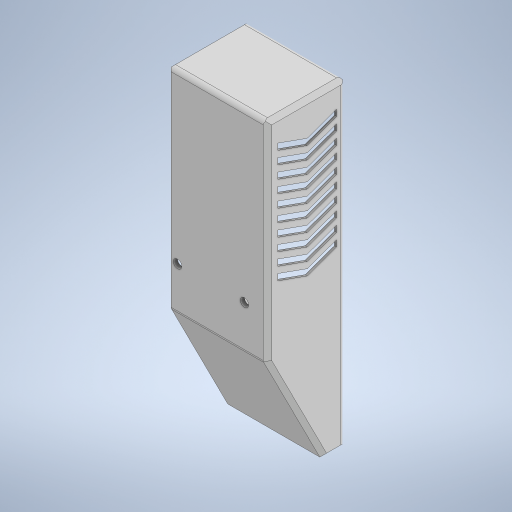
# Autodesk Inventor part: LewyBłotnik
Saved by Autodesk Inventor 2024 (Build 280153000, 153)
## iProperties
Created: 2025-05-22
Part Number: LewyBłotnik
Material: Ogólny
Document SubType Name: Modeling
Designer: Victoria
Density: 1 g/cm^3
Appearance: Domyślna
Author: Victoria
Autodesk Inventor part; units mm, degrees
ref_plane "YZ Plane" through (0, 0, 0) normal (1, 0, 0) x (0, 1, 0)
ref_plane "XZ Plane" through (0, 0, 0) normal (0, 1, 0) x (-1, 0, 0)
ref_plane "XY Plane" through (0, 0, 0) normal (0, 0, 1) x (1, 0, 0)
sketch "Szkic1" plane through (0, 0, 0) normal (0, 0, 1) x (1, 0, 0)
  circle A0 centre (16, 0) radius 2
  circle A1 centre (-16, 0) radius 2
  line L0 (28, -73) -> (-21, -73)
  line L1 (-21, -73) -> (-21, 0)
  line L2 (28, 80) -> (-21, 80)
  line L3 (-21, 80) -> (-21, 0)
  line L4 (28, -73) -> (27, -73)
  line L5 (27, -73) -> (27, 80)
  point P0 (0, 0)
  point P1 (-21, 83.4616)
  dimension "d0" = 4
  dimension "d48" = 1
  constraints: 12 end point, 3 perpendicular, 3 point on line, 2 centre point
  measures "d0" diameter of A0
  measures "d48" distance of L0.start L4.end
extrude "Wyciągnięcie proste1" add sketch "Szkic1" along normal blind 2
sketch "Szkic2" plane through (0, 0, 0) normal (0, 0, -1) x (-1, 0, 0)
  line L0 (21, -73) -> (-27, -73) projected
  line L1 (21, 80) -> (21, -73) projected
  circle A0 centre (16, 0) radius 2 projected
  circle A1 centre (-16, 0) radius 2 projected
  line L2 (19, -10) -> (21, -10)
  line L3 (-27, 80) -> (21, 80) projected
  line L4 (19, -71) -> (-26, -71)
  line L5 (-26, -71) -> (-26, 78)
  line L6 (-26, 78) -> (19, 78)
  line L7 (19, 78) -> (19, -71)
  line L8 (19, 68) -> (21, 68)
  line L9 (-27, -73) -> (-27, 80) projected
  point P0 (0, 0)
  dimension "d10" = 2
  constraints: 12 end point, 3 point on line, 2 perpendicular, 1 other
  measures "d10" distance between parallel lines of L1 L7
extrude "Wyciągnięcie proste2" add sketch "Szkic2" along normal blind 35 contours L0 L9 L3 L1 L8 L7 L6 L5 L4 L2 | L2 L7 L8 L1
sketch "Szkic7" plane through (27, -73, 2) normal (1, 0, 0) x (0, 0, -1)
  line L0 (0, 0) -> (0, 153) projected
  line L1 (37, 0) -> (0, 0) projected
  line L2 (0, 53) -> (27, 0) projected
  point P0 (2, 73)
extrude "Wyciągnięcie proste7" cut sketch "Szkic7" against normal up to surface (48 mm away)
sketch "Szkic9" plane through (27, -73, -35) normal (1, 0, 0) x (0, 0, -1)
  line L0 (-37, 53) -> (-10, 0) projected
  line L1 (0, 0) -> (-10, 0) projected
  line L2 (0, 153) -> (0, 0) projected
  line L3 (0, 153) -> (-37, 153) projected
  line L4 (-37, 53) -> (-37, 153) projected
  line L5 (-10, 0) -> (-8, 0)
  line L6 (0, 0) -> (-10, 0) projected
  line L7 (-37, 53) -> (-35, 53)
  line L8 (-35, 53) -> (-8, 0)
  point P0 (-35, 73)
  point P1 (-8, 0)
  dimension "d54" = 2
  dimension "d55" = 2
  constraints: 6 end point, 1 horizontal, 1 point on line
  measures "d54" distance of L0.end L5.end
  measures "d55" distance of L0.start L7.end
extrude "Wyciągnięcie proste9" add sketch "Szkic9" against normal up to surface (48 mm away) contours L7 L8 L1 L0
chamfer "Faza2" distance 2 angle 45 16 edges at (27, -46.5, -11.5) (27, -73, -30) (27, 30, 2) (27, 80, -16.5) (26, -45.5, -12.9906) (26, -71, -30.4906) (26, 29, 0) (26, 78, -17.5) (-21, -46.5, -11.5) (-21, -73, -30) (-21, 30, 2) (-21, 80, -16.5) (-19, 29, 0) (-19, -45.5, -12.9906) (-19, -71, -30.4906) (-19, 78, -17.5)
fillet "Zaokrąglenie2" radius 2 6 edges at (3, -73, -35) (3, 80, -35) (-21, 3.5, -35) (27, 3.5, -35) (3, -20, 2) (3, 80, 2)
sketch "Szkic13" plane through (27, -19.5199, 0) normal (1, 0, 0) x (0, 0, -1)
  line L0 (33, 97.5199) -> (33, 106.5199)
  line L1 (33, 106.5199) -> (17, 106.5199)
  line L2 (1, 106.5199) -> (33, 106.5199)
  line L3 (17, 106.5199) -> (17, 193.3833)
  line L4 (17, 106.5199) -> (17, 111.5199)
  line L5 (31, 106.5199) -> (17, 111.5199)
  line L6 (17, 111.5199) -> (3, 106.5199)
  line L7 (31, 106.5199) -> (31, 109.5199)
  line L8 (17, 111.5199) -> (17, 114.5199)
  line L9 (17, 114.5199) -> (31, 109.5199)
  line L10 (3, 106.5199) -> (3, 109.5199)
  line L11 (3, 193.7998) -> (3, 99.5199)
  line L12 (3, 109.5199) -> (17, 114.5199)
  line L13 (17, 117.5199) -> (3, 112.5199)
  line L14 (3, 115.5199) -> (17, 120.5199)
  line L15 (3, 112.5199) -> (3, 115.5199)
  line L16 (31, 112.5199) -> (17, 117.5199)
  line L17 (17, 120.5199) -> (31, 115.5199)
  line L18 (31, 112.5199) -> (31, 115.5199)
  line L19 (17, 123.5199) -> (3, 118.5199)
  line L20 (3, 121.5199) -> (17, 126.5199)
  line L21 (3, 118.5199) -> (3, 121.5199)
  line L22 (31, 118.5199) -> (17, 123.5199)
  line L23 (17, 126.5199) -> (31, 121.5199)
  line L24 (31, 118.5199) -> (31, 121.5199)
  line L25 (17, 129.5199) -> (3, 124.5199)
  line L26 (3, 127.5199) -> (17, 132.5199)
  line L27 (3, 124.5199) -> (3, 127.5199)
  line L28 (31, 124.5199) -> (17, 129.5199)
  line L29 (17, 132.5199) -> (31, 127.5199)
  line L30 (31, 124.5199) -> (31, 127.5199)
  line L31 (17, 135.5199) -> (3, 130.5199)
  line L32 (3, 133.5199) -> (17, 138.5199)
  line L33 (3, 130.5199) -> (3, 133.5199)
  line L34 (31, 130.5199) -> (17, 135.5199)
  line L35 (17, 138.5199) -> (31, 133.5199)
  line L36 (31, 130.5199) -> (31, 133.5199)
  line L37 (17, 141.5199) -> (3, 136.5199)
  line L38 (3, 139.5199) -> (17, 144.5199)
  line L39 (3, 136.5199) -> (3, 139.5199)
  line L40 (31, 136.5199) -> (17, 141.5199)
  line L41 (17, 144.5199) -> (31, 139.5199)
  line L42 (31, 136.5199) -> (31, 139.5199)
  line L43 (17, 147.5199) -> (3, 142.5199)
  line L44 (3, 145.5199) -> (17, 150.5199)
  line L45 (3, 142.5199) -> (3, 145.5199)
  line L46 (31, 142.5199) -> (17, 147.5199)
  line L47 (17, 150.5199) -> (31, 145.5199)
  line L48 (31, 142.5199) -> (31, 145.5199)
  line L49 (17, 153.5199) -> (3, 148.5199)
  line L50 (3, 151.5199) -> (17, 156.5199)
  line L51 (3, 148.5199) -> (3, 151.5199)
  line L52 (31, 148.5199) -> (17, 153.5199)
  line L53 (17, 156.5199) -> (31, 151.5199)
  line L54 (31, 148.5199) -> (31, 151.5199)
  line L55 (17, 159.5199) -> (3, 154.5199)
  line L56 (3, 157.5199) -> (17, 162.5199)
  line L57 (3, 154.5199) -> (3, 157.5199)
  line L58 (31, 154.5199) -> (17, 159.5199)
  line L59 (17, 162.5199) -> (31, 157.5199)
  line L60 (31, 154.5199) -> (31, 157.5199)
  line L61 (17, 165.5199) -> (3, 160.5199)
  line L62 (3, 163.5199) -> (17, 168.5199)
  line L63 (3, 160.5199) -> (3, 163.5199)
  line L64 (31, 160.5199) -> (17, 165.5199)
  line L65 (17, 168.5199) -> (31, 163.5199)
  line L66 (31, 160.5199) -> (31, 163.5199)
  line L67 (33, 97.5199) -> (33, -51.4801) projected
  line L68 (0, 97.5199) -> (33, 97.5199) projected
  line L69 (0, 0) -> (0, 97.5199) projected
  line L70 (26.2257, -51.4801) -> (0, 0) projected
  line L71 (33, -51.4801) -> (26.2257, -51.4801) projected
  line L72 (3, 88.5199) -> (3, 85.5199)
  line L73 (1, 88.5199) -> (33, 88.5199)
  line L74 (33, 88.5199) -> (17, 88.5199)
  line L75 (33, 97.5199) -> (33, 88.5199)
  line L76 (31, 70.5199) -> (31, 67.5199)
  line L77 (31, 70.5199) -> (17, 65.5199)
  line L78 (17, 62.5199) -> (31, 67.5199)
  line L79 (31, 64.5199) -> (31, 61.5199)
  line L80 (31, 64.5199) -> (17, 59.5199)
  line L81 (31, 58.5199) -> (31, 55.5199)
  line L82 (17, 56.5199) -> (31, 61.5199)
  line L83 (31, 58.5199) -> (17, 53.5199)
  line L84 (17, 88.5199) -> (17, 83.5199)
  line L85 (31, 88.5199) -> (17, 83.5199)
  line L86 (31, 88.5199) -> (31, 85.5199)
  line L87 (17, 68.5199) -> (31, 73.5199)
  line L88 (31, 76.5199) -> (17, 71.5199)
  line L89 (31, 76.5199) -> (31, 73.5199)
  line L90 (17, 74.5199) -> (31, 79.5199)
  line L91 (31, 82.5199) -> (17, 77.5199)
  line L92 (17, 83.5199) -> (17, 80.5199)
  line L93 (17, 80.5199) -> (31, 85.5199)
  line L94 (31, 82.5199) -> (31, 79.5199)
  line L95 (17, 83.5199) -> (3, 88.5199)
  line L96 (3, 85.5199) -> (17, 80.5199)
  line L97 (17, 77.5199) -> (3, 82.5199)
  line L98 (3, 79.5199) -> (17, 74.5199)
  line L99 (17, 71.5199) -> (3, 76.5199)
  line L100 (3, 73.5199) -> (17, 68.5199)
  line L101 (17, 65.5199) -> (3, 70.5199)
  line L102 (17, 47.5199) -> (3, 52.5199)
  line L103 (17, 53.5199) -> (3, 58.5199)
  line L104 (3, 61.5199) -> (17, 56.5199)
  line L105 (17, 59.5199) -> (3, 64.5199)
  line L106 (3, 67.5199) -> (17, 62.5199)
  line L107 (3, 55.5199) -> (17, 50.5199)
  line L108 (3, 49.5199) -> (17, 44.5199)
  line L109 (3, 46.5199) -> (3, 43.5199)
  line L110 (17, 41.5199) -> (3, 46.5199)
  line L111 (3, 43.5199) -> (17, 38.5199)
  line L112 (3, 40.5199) -> (3, 37.5199)
  line L113 (17, 35.5199) -> (3, 40.5199)
  line L114 (3, 37.5199) -> (17, 32.5199)
  line L115 (3, 82.5199) -> (3, 79.5199)
  line L116 (3, 76.5199) -> (3, 73.5199)
  line L117 (3, 70.5199) -> (3, 67.5199)
  line L118 (3, 64.5199) -> (3, 61.5199)
  line L119 (3, 58.5199) -> (3, 55.5199)
  line L120 (3, 1.24) -> (3, 95.5199)
  line L121 (17, 88.5199) -> (17, 1.6565)
  line L122 (3, 52.5199) -> (3, 49.5199)
  line L123 (17, 50.5199) -> (31, 55.5199)
  line L124 (31, 52.5199) -> (31, 49.5199)
  line L125 (31, 52.5199) -> (17, 47.5199)
  line L126 (17, 44.5199) -> (31, 49.5199)
  line L127 (31, 46.5199) -> (31, 43.5199)
  line L128 (31, 46.5199) -> (17, 41.5199)
  line L129 (17, 38.5199) -> (31, 43.5199)
  line L130 (31, 40.5199) -> (31, 37.5199)
  line L131 (17, 32.5199) -> (31, 37.5199)
  line L132 (31, 40.5199) -> (17, 35.5199)
  line L133 (3, 34.5199) -> (3, 31.5199)
  line L134 (31, 34.5199) -> (31, 31.5199)
  line L135 (17, 29.5199) -> (3, 34.5199)
  line L136 (3, 31.5199) -> (17, 26.5199)
  line L137 (17, 26.5199) -> (31, 31.5199)
  line L138 (31, 34.5199) -> (17, 29.5199)
  point P0 (0, 19.5199)
  point P1 (0, 174.5199)
  point P2 (1, 106.5199)
  point P3 (3, 99.5199)
  point P4 (-38.868, 30.6038)
  point P5 (3, 202.1317)
  point P6 (1, 88.5199)
  point P7 (3, -7.0919)
  point P8 (0, 20.5199)
  dimension "d85" = 16
  dimension "d86" = 5
  dimension "d87" = 3
  dimension "d88" = 3
  dimension "d89" = 3
  dimension "d90" = 6
  constraints: 264 end point, 79 symmetric about line, 10 point on line, 1 midpoint, 1 perpendicular, 1 vertical, 125 other
  measures "d85" distance of L2.end L1.end
  measures "d86" distance of L1.end L4.end
  measures "d87" distance of L5.start L7.end
  measures "d88" distance of L4.end L8.end
  measures "d89" distance of L10.start L10.end
  measures "d90" distance of L4.end L16.end
extrude "Wyciągnięcie proste13" cut sketch "Szkic13" against normal blind 10 contours L95 L92 L96 L72 | L85 L86 L93 L92 | L97 L121 L98 L115 | L91 L94 L90 L121 | L99 L121 L100 L116 | L88 L89 L87 L121 | L101 L121 L106 L117 | L77 L76 L78 L121 | L105 L121 L104 L118 | L80 L79 L82 L121 | L103 L121 L107 L119 | L83 L81 L123 L121 | L102 L121 L108 L120 | L125 L124 L126 L121 | L110 L121 L111 L109 | L128 L127 L129 L121 | L113 L121 L114 L112 | L132 L130 L131 L121 | L135 L121 L136 L120 | L138 L134 L137 L121
sketch "Szkic14" plane through (-21, -19.5199, 0) normal (-1, 0, 0) x (0, 0, 1)
  line L0 (1.4142, 98.9341) -> (0, 97.5199) projected
  line L1 (-35, 95.5199) -> (-35, -49.4801) projected
  line L2 (0, 97.5199) -> (-35, 97.5199)
  line L3 (-35, 97.5199) -> (-35, 9.5199)
  line L4 (-35, 9.5199) -> (0, 9.5199)
  line L5 (0, 9.5199) -> (0, 97.5199)
  point P0 (0, 19.5199)
  dimension "d94" = 88
  constraints: 8 end point, 2 parallel, 1 horizontal, 1 perpendicular, 1 point on line
  measures "d94" distance of L3.end L2.end
extrude "Wyciągnięcie proste14" cut sketch "Szkic14" against normal blind 10
